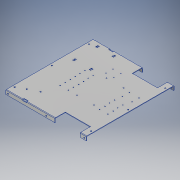
# Autodesk Inventor part: BellyPan2
Saved by Autodesk Inventor 2016 (Build 200138000, 138)
## iProperties
Created: 2017-01-21
Part Number: BellyPan2
Material: Aluminum 6061
Document SubType Name: Modeling
Designer: hamblettk
Density: 2.7 g/cm^3
Appearance: Aluminum - Flat
Author: hamblettk
Autodesk Inventor part; units mm, degrees
ref_plane "YZ Plane" through (0, 0, 0) normal (1, 0, 0) x (0, 1, 0)
ref_plane "XZ Plane" through (0, 0, 0) normal (0, 1, 0) x (-1, 0, 0)
ref_plane "XY Plane" through (0, 0, 0) normal (0, 0, 1) x (1, 0, 0)
sketch "Sketch1" plane through (0, 0, 0) normal (0, 1, 0) x (-1, 0, 0)
  line L0 (0, 0) -> (495.3, 0)
  line L1 (495.3, 0) -> (495.3, -539.75)
  line L2 (495.3, -539.75) -> (0, -539.75)
  line L3 (0, -539.75) -> (0, 0)
  dimension "d0" = 495.3
  dimension "d1" = 539.75
  constraints: 8 end point, 2 parallel, 1 horizontal, 1 perpendicular
  measures "d0" distance of L1.end L2.end
  measures "d1" distance of L0.end L1.end
extrude "Extrusion1" add sketch "Sketch1" along normal blind 3.175
sketch "Sketch2" plane through (0, 0, 0) normal (1, 0, 0) x (0, 0, -1)
  line L0 (0, 3.175) -> (0, 15.875)
  line L1 (0, 15.875) -> (3.175, 15.875)
  line L2 (3.175, 15.875) -> (3.175, 3.175)
  line L3 (0, 3.175) -> (539.75, 3.175) projected
  line L4 (3.175, 3.175) -> (0, 3.175)
  line L5 (539.75, 3.175) -> (539.75, 15.875)
  line L6 (539.75, 15.875) -> (536.575, 15.875)
  line L7 (536.575, 15.875) -> (536.575, 3.175)
  line L8 (539.75, 0) -> (539.75, 3.175) projected
  line L9 (536.575, 3.175) -> (539.75, 3.175)
  point P0 (0, 0)
  dimension "d4" = 12.7
  dimension "d5" = 3.175
  dimension "d6" = 12.7
  dimension "d7" = 3.175
  constraints: 16 end point, 5 perpendicular, 2 vertical, 1 horizontal, 1 point on line
  measures "d4" distance of L0.start L0.end
  measures "d5" distance of L0.end L1.end
  measures "d6" distance of L3.end L5.end
  measures "d7" distance of L5.end L6.end
extrude "Extrusion2" add sketch "Sketch2" against normal blind 495.3
fillet "Fillet1" radius 3.175 4 edges at (-247.65, 3.175, -536.575) (-247.65, 3.175, -3.175) (-247.65, 0, 0) (-247.65, 0, -539.75)
sketch "Sketch3" plane through (-495.3, 15.875, -539.75) normal (0, 1, 0) x (1, 0, 0)
  line L0 (495.3, 0) -> (0, 0) projected
  line L1 (495.3, 0) -> (457.2, 0)
  line L2 (457.2, 0) -> (304.8, 0)
  line L3 (304.8, 0) -> (304.8, -50.8)
  line L4 (304.8, -50.8) -> (457.2, -50.8)
  line L5 (457.2, -50.8) -> (457.2, 0)
  line L6 (0, -6.35) -> (0, -533.4) projected
  line L7 (0, -269.875) -> (495.3, -269.875)
  line L8 (495.3, -539.75) -> (0, -539.75)
  line L9 (457.2, -539.75) -> (304.8, -539.75)
  line L10 (304.8, -539.75) -> (304.8, -488.95)
  line L11 (304.8, -488.95) -> (457.2, -488.95)
  line L12 (457.2, -488.95) -> (457.2, -539.75)
  point P0 (495.3, -539.75)
  dimension "d11" = 38.1
  dimension "d12" = 152.4
  dimension "d13" = 50.8
  constraints: 22 end point, 6 symmetric about line, 4 point on line, 2 horizontal, 1 midpoint, 1 perpendicular, 1 vertical
  measures "d11" distance of L0.start L1.end
  measures "d12" distance of L1.end L2.end
  measures "d13" distance of L2.end L3.end
extrude "Extrusion3" cut sketch "Sketch3" against normal blind 495.3
sketch "Sketch5" plane through (-495.3, 15.875, -3.175) normal (0, 1, 0) x (1, 0, 0)
  line L0 (304.8, -3.175) -> (304.8, 0) projected
  line L1 (304.8, 0) -> (0, 0) projected
  line L2 (0, -3.175) -> (0, 0) projected
  line L3 (304.8, -3.175) -> (0, -3.175) projected
  line L4 (457.2, 0) -> (457.2, -3.175) projected
  line L5 (495.3, -3.175) -> (457.2, -3.175) projected
  line L6 (495.3, 0) -> (495.3, -3.175) projected
  line L7 (495.3, 0) -> (457.2, 0) projected
  line L8 (457.2, 536.575) -> (457.2, 533.4) projected
  line L9 (495.3, 533.4) -> (457.2, 533.4) projected
  line L10 (495.3, 536.575) -> (495.3, 533.4) projected
  line L11 (495.3, 536.575) -> (457.2, 536.575) projected
  line L12 (304.8, 533.4) -> (304.8, 536.575) projected
  line L13 (304.8, 536.575) -> (0, 536.575) projected
  line L14 (0, 533.4) -> (0, 536.575) projected
  line L15 (304.8, 533.4) -> (0, 533.4) projected
extrude "Extrusion4" add sketch "Sketch5" along normal blind 9.525
sketch "Sketch6" plane through (-190.5, 0, -50.8) normal (1, 0, 0) x (0, 0, -1)
  line L0 (0, 0) -> (-47.625, 0) projected
  line L1 (0, 3.175) -> (0, 0) projected
  line L2 (-44.45, 3.175) -> (0, 3.175) projected
  arc A0 (-47.625, 6.35) -> (-44.45, 3.175) centre (-44.45, 6.35) ccw projected
  line L3 (-47.625, 25.4) -> (-47.625, 6.35) projected
  line L4 (-50.8, 25.4) -> (-47.625, 25.4) projected
  line L5 (-50.8, 3.175) -> (-50.8, 25.4) projected
  arc A1 (-50.8, 3.175) -> (-47.625, 0) centre (-47.625, 3.175) ccw projected
  line L6 (485.775, 0) -> (438.15, 0) projected
  arc A2 (485.775, 0) -> (488.95, 3.175) centre (485.775, 3.175) ccw projected
  line L7 (488.95, 25.4) -> (488.95, 3.175) projected
  line L8 (485.775, 25.4) -> (488.95, 25.4) projected
  line L9 (485.775, 6.35) -> (485.775, 25.4) projected
  arc A3 (482.6, 3.175) -> (485.775, 6.35) centre (482.6, 6.35) ccw projected
  line L10 (438.15, 3.175) -> (482.6, 3.175) projected
  line L11 (438.15, 3.175) -> (438.15, 0) projected
  point P0 (-50.8, 0)
extrude "Extrusion5" cut sketch "Sketch6" against normal blind 3.175
sketch "Sketch7" plane through (-495.3, 6.35, -536.575) normal (0, 0, 1) x (1, 0, 0)
  line L0 (301.625, 0) -> (301.625, 19.05) projected
  line L1 (301.625, 9.525) -> (247.65, 9.525)
  circle A0 centre (247.65, 9.525) radius 3.5687
  point P0 (495.3, -6.35)
  dimension "d21" = 7.1374
  dimension "d22" = 53.975
  constraints: 2 end point, 1 centre point, 1 coincident, 1 horizontal, 1 midpoint
  measures "d21" diameter of A0
  measures "d22" distance from line of L0 L1.end
extrude "Extrusion6" cut sketch "Sketch7" against normal blind 3.175
sketch "Sketch8" plane through (-495.3, 6.35, -3.175) normal (0, 0, -1) x (-1, 0, 0)
  line L0 (-301.625, 19.05) -> (-301.625, 0) projected
  circle A0 centre (-247.65, 9.525) radius 3.5687
  point P0 (-495.3, -6.35)
  dimension "d26" = 7.1374
  constraints: 1 centre point
  measures "d26" diameter of A0
extrude "Extrusion7" cut sketch "Sketch8" against normal blind 3.175
sketch "Sketch9" plane through (-495.3, 6.35, -536.575) normal (0, 0, 1) x (1, 0, 0)
  line L0 (0, 0) -> (0, 19.05) projected
  line L1 (0, 9.525) -> (12.7, 9.525)
  circle A0 centre (12.7, 9.525) radius 3.5687
  point P0 (495.3, -6.35)
  dimension "d29" = 12.7
  dimension "d30" = 7.1374
  constraints: 2 end point, 1 centre point, 1 coincident, 1 horizontal, 1 midpoint
  measures "d29" distance of L1.start L1.end
  measures "d30" diameter of A0
extrude "Extrusion8" cut sketch "Sketch9" against normal blind 3.175
sketch "Sketch10" plane through (-495.3, 6.35, -3.175) normal (0, 0, -1) x (-1, 0, 0)
  line L0 (0, 0) -> (0, 19.05) projected
  line L1 (0, 9.525) -> (-12.7, 9.525)
  circle A0 centre (-12.7, 9.525) radius 3.5687
  point P0 (-495.3, -6.35)
  dimension "d33" = 12.7
  dimension "d34" = 7.1374
  constraints: 2 end point, 1 centre point, 1 coincident, 1 horizontal, 1 midpoint
  measures "d33" distance of L1.start L1.end
  measures "d34" diameter of A0
extrude "Extrusion9" cut sketch "Sketch10" against normal blind 3.175
sketch "Sketch11" plane through (0, 6.35, -3.175) normal (0, 0, -1) x (-1, 0, 0)
  line L0 (0, 0) -> (0, 19.05) projected
  line L1 (0, 9.525) -> (12.7, 9.525)
  circle A0 centre (12.7, 9.525) radius 3.5687
  point P0 (0, -6.35)
  dimension "d37" = 12.7
  dimension "d38" = 7.1374
  constraints: 2 end point, 1 centre point, 1 coincident, 1 horizontal, 1 midpoint
  measures "d37" distance of L1.start L1.end
  measures "d38" diameter of A0
extrude "Extrusion10" cut sketch "Sketch11" against normal blind 3.175
sketch "Sketch12" plane through (-38.1, 6.35, -536.575) normal (0, 0, 1) x (1, 0, 0)
  line L0 (38.1, 0) -> (0, 0) projected
  line L1 (38.1, 19.05) -> (38.1, 0) projected
  point P0 (38.1, -6.35)
  point P1 (25.3992, 9.525)
  dimension "d41" = 9.525
  dimension "d42" = 12.7008
  measures "d41" distance from line of L0 point (25.399, 9.525)
  measures "d42" distance from line of L1 point (25.399, 9.525)
hole "Hole1" at (-12.7008, 15.875, -536.575) direction (0, 0, -1) diameter 7.1374 end through all
sketch "Sketch15" plane through (0, 0, 0) normal (0, -1, 0) x (1, 0, 0)
  line L0 (-495.3, -3.175) -> (-495.3, 0) projected
  line L1 (-495.3, 0) -> (-380.1364, 0)
  line L2 (-495.3, 0) -> (-193.675, 0) projected
  line L3 (-380.1364, 0) -> (-367.4364, 0)
  line L4 (-380.1364, 0) -> (-392.8364, 0)
  line L5 (-392.8364, 0) -> (-392.8364, -9.525)
  line L6 (-392.8364, -9.525) -> (-367.4364, -9.525)
  line L7 (-367.4364, -9.525) -> (-367.4364, 0)
  line L8 (-495.3, -533.4) -> (-495.3, -6.35) projected
  line L9 (-495.3, -269.875) -> (0, -269.875)
  line L10 (-495.3, -539.75) -> (-380.1364, -539.75)
  line L11 (-495.3, -539.75) -> (-193.675, -539.75)
  line L12 (-392.8364, -539.75) -> (-392.8364, -530.225)
  line L13 (-392.8364, -530.225) -> (-367.4364, -530.225)
  line L14 (-367.4364, -530.225) -> (-367.4364, -539.75)
  point P0 (0, 0)
  dimension "d56" = 115.1636
  dimension "d57" = 12.7
  dimension "d58" = 12.7
  dimension "d59" = 9.525
  constraints: 24 end point, 7 symmetric about line, 6 point on line, 3 perpendicular, 1 horizontal, 1 midpoint
  measures "d56" distance of L0.end L1.end
  measures "d57" distance of L1.end L3.end
  measures "d58" distance of L1.end L4.end
  measures "d59" distance of L4.end L5.end
extrude "Extrusion11" cut sketch "Sketch15" against normal blind 3.175
sketch "Sketch16" plane through (0, 0, 0) normal (0, -1, 0) x (1, 0, 0)
  circle A0 centre (-12.7, -269.875) radius 3.5687
  line L0 (0, -536.575) -> (0, -3.175) projected
  line L1 (-38.1, -539.75) -> (0, -539.75) projected
  circle A1 centre (-12.7, -498.475) radius 3.5687
  circle A2 centre (-12.7, -41.275) radius 3.5687
  circle A3 centre (-482.6, -269.875) radius 3.5687
  line L2 (-495.3, -3.175) -> (-495.3, -536.575) projected
  line L3 (-495.3, -539.75) -> (-392.8364, -539.75) projected
  circle A4 centre (-482.6, -498.475) radius 3.5687
  circle A5 centre (-482.6, -41.275) radius 3.5687
  point P0 (0, 0)
  dimension "d62" = 7.1374
  dimension "d63" = 12.7
  dimension "d64" = 269.875
  dimension "d65" = 7.1374
  dimension "d66" = 12.7
  dimension "d67" = 228.6
  dimension "d68" = 7.1374
  dimension "d69" = 12.7
  dimension "d70" = 228.6
  dimension "d71" = 7.1374
  dimension "d72" = 12.7
  dimension "d73" = 269.875
  dimension "d74" = 7.1374
  dimension "d75" = 12.7
  dimension "d76" = 228.6
  dimension "d77" = 7.1374
  dimension "d78" = 12.7
  dimension "d79" = 228.6
  constraints: 6 centre point
  measures "d62" diameter of A0
  measures "d63" distance from line of L0 A0.centre
  measures "d64" distance from line of L1 A0.centre
  measures "d65" diameter of A1
  measures "d66" distance from line of L0 A1.centre
  measures "d67" distance of A0.centre A1.centre
  measures "d68" diameter of A2
  measures "d69" distance from line of L0 A2.centre
  measures "d70" distance of A0.centre A2.centre
  measures "d71" diameter of A3
  measures "d72" distance from line of L2 A3.centre
  measures "d73" distance from line of L3 A3.centre
  measures "d74" diameter of A4
  measures "d75" distance from line of L2 A4.centre
  measures "d76" distance of A3.centre A4.centre
  measures "d77" diameter of A5
  measures "d78" distance from line of L2 A5.centre
  measures "d79" distance of A3.centre A5.centre
extrude "Extrusion12" cut sketch "Sketch16" against normal blind 3.175
sketch "Sketch18" plane through (0, 3.175, 0) normal (0, -1, 0) x (1, 0, 0)
  line L0 (-392.8364, -533.4) -> (-367.4364, -533.4) projected
  line L1 (-392.8364, -539.75) -> (-392.8364, -533.4) projected
  line L2 (-392.8364, -539.75) -> (-367.4364, -539.75) projected
  line L3 (-367.4364, -533.4) -> (-367.4364, -539.75) projected
  line L4 (-367.4364, -6.35) -> (-392.8364, -6.35) projected
  line L5 (-367.4364, 0) -> (-367.4364, -6.35) projected
  line L6 (-367.4364, 0) -> (-392.8364, 0) projected
  line L7 (-392.8364, -6.35) -> (-392.8364, 0) projected
  point P0 (0, 0)
extrude "Extrusion13" cut sketch "Sketch18" against normal blind 3.175
sketch "Sketch19" plane through (-193.675, 0, -50.8) normal (0, 0, 1) x (1, 0, 0)
  line L0 (155.575, 0) -> (0, 0) projected
  line L1 (155.575, 3.175) -> (155.575, 0) projected
  line L2 (0, 3.175) -> (155.575, 3.175) projected
  line L3 (0, 3.175) -> (0, 0) projected
  point P0 (193.675, 0)
extrude "Extrusion14" cut sketch "Sketch19" against normal blind 12.7
sketch "Sketch20" plane through (-38.1, 0, -488.95) normal (0, 0, -1) x (-1, 0, 0)
  line L0 (155.575, 0) -> (0, 0) projected
  line L1 (155.575, 0) -> (155.575, 3.175) projected
  line L2 (0, 3.175) -> (155.575, 3.175) projected
  line L3 (0, 3.175) -> (0, 0) projected
  point P0 (-38.1, 0)
extrude "Extrusion15" cut sketch "Sketch20" against normal blind 12.7
sketch "Sketch21" plane through (0, 0, 0) normal (0, -1, 0) x (1, 0, 0)
  circle A0 centre (-350.8851, -350.2396) radius 2.2497
  circle A1 centre (-350.9114, -319.1371) radius 2.2497
  circle A2 centre (-350.938, -287.5981) radius 2.2497
  ellipse E0 centre (-354.1933, -225.6154) end of major axis (-352.0021, -225.6135) minor radius 2.1905
  ellipse E1 centre (-354.2089, -194.5782) end of major axis (-352.0176, -194.5764) minor radius 2.1899
  ellipse E2 centre (-303.4089, -194.5392) end of major axis (-301.2176, -194.5374) minor radius 2.1899
  ellipse E3 centre (-303.3933, -225.5744) end of major axis (-301.2021, -225.5726) minor radius 2.1905
  ellipse E4 centre (-300.1641, -256.8149) end of major axis (-302.6771, -256.817) minor radius 2.5126
  circle A3 centre (-300.138, -287.5552) radius 2.513
  circle A4 centre (-300.1114, -319.0942) radius 2.513
  circle A5 centre (-300.0851, -350.1948) radius 2.513
  circle A6 centre (-350.8851, -350.2396) radius 2.513
  circle A7 centre (-350.9114, -319.1371) radius 2.413
  circle A8 centre (-350.938, -287.5981) radius 2.513
  ellipse E5 centre (-350.9641, -256.8541) end of major axis (-348.5511, -256.8521) minor radius 2.4126
  circle A9 centre (-246.6296, -350.841) radius 2.667
  circle A10 centre (-246.9059, -168.5708) radius 2.667
  circle A11 centre (-142.512, -168.4126) radius 2.667
  circle A12 centre (-142.2357, -350.6828) radius 2.667
  ellipse E6 centre (-101.9617, -356.43) end of major axis (-104.3747, -356.43) minor radius 2.413
  ellipse E7 centre (-51.1617, -356.43) end of major axis (-53.5747, -356.43) minor radius 2.413
  ellipse E8 centre (-51.1617, -323.2691) end of major axis (-53.5747, -323.2691) minor radius 2.413
  ellipse E9 centre (-101.9617, -323.2691) end of major axis (-104.3747, -323.2691) minor radius 2.413
  ellipse E10 centre (-105.1502, -292.1816) end of major axis (-107.3414, -292.1816) minor radius 2.1913
  ellipse E11 centre (-105.1502, -261.0646) end of major axis (-107.3414, -261.0646) minor radius 2.1913
  ellipse E12 centre (-54.3502, -292.1816) end of major axis (-56.5414, -292.1816) minor radius 2.1913
  ellipse E13 centre (-54.3502, -261.0646) end of major axis (-56.5414, -261.0646) minor radius 2.1913
  circle A13 centre (-42.4909, -216.236) radius 2.5
  circle A14 centre (-101.1909, -216.2459) radius 2.5
  circle A15 centre (-100.642, -173.7423) radius 2.5
  circle A16 centre (-41.942, -173.7324) radius 2.5
  circle A17 centre (-275.3803, -143.6352) radius 1.905
  circle A18 centre (-227.6284, -143.5398) radius 1.905
  circle A19 centre (-227.7168, -100.4868) radius 1.905
  circle A20 centre (-275.4663, -100.5823) radius 1.905
  ellipse E14 centre (-434.736, -472.3219) end of major axis (-438.165, -472.3219) minor radius 3.429
  ellipse E15 centre (-377.586, -444.3819) end of major axis (-374.157, -444.3819) minor radius 3.429
  circle A21 centre (-12.6998, -269.8753) radius 3.5687
  circle A22 centre (-12.6998, -498.4753) radius 3.5685
  circle A23 centre (-12.6998, -41.2753) radius 3.5687
  line L0 (-438.5985, -28.3241) -> (-448.6768, -28.3241)
  line L1 (-448.6768, -28.3241) -> (-448.6768, -35.0231)
  spline S0 degree 4 poles (-448.6768, -35.0231) (-448.6639, -35.1127) (-448.348, -35.761) (-448.3812, -35.7746) (-448.1019, -36.3268) (-448.1852, -36.1139) (-448.2253, -36.0497) (-448.2684, -35.9471) (-448.3123, -35.8601) (-448.3471, -35.7301) (-448.3902, -35.6264) (-448.4102, -35.543) (-448.4284, -35.4842) knots 0 0 0 0 0 0.320714 0.419759 0.501148 0.569271 0.635606 0.702263 0.768643 0.834806 1 1 1 1 1
  line L2 (-448.4284, -35.4842) -> (-438.847, -35.4842)
  spline S1 degree 4 poles (-438.847, -35.4842) (-438.8355, -35.6171) (-438.8088, -35.8104) (-438.7923, -36.0459) (-438.74, -36.3561) (-438.7353, -36.5543) (-438.7189, -36.7533) (-438.7047, -36.966) (-438.6926, -37.1615) (-438.649, -37.7375) (-438.6347, -34.9543) (-438.603, -36.3425) (-438.5985, -35.0231) knots 0 0 0 0 0 0.176534 0.246794 0.316361 0.385081 0.452716 0.516863 0.592826 0.686487 1 1 1 1 1
  line L3 (-438.5985, -35.0231) -> (-438.5985, -28.3241)
  line L4 (-448.352, -20.7549) -> (-438.5985, -20.7549)
  line L5 (-448.352, -23.9299) -> (-448.352, -20.7549)
  line L6 (-438.5985, -23.9299) -> (-448.352, -23.9299)
  line L7 (-438.5985, -20.7549) -> (-438.5985, -23.9299)
  line L8 (-337.0695, -35.4845) -> (-347.0864, -35.4845)
  line L9 (-347.0864, -35.4845) -> (-347.0864, -28.3951)
  line L10 (-346.8284, -35.4842) -> (-337.247, -35.4842)
  line L11 (-337.0695, -28.3951) -> (-337.0695, -35.4845)
  ellipse E16 centre (-337.324, -28.3952) end of major axis (-337.5783, -28.3952) minor radius 0.0044 (-337.0698, -28.3951) -> (-337.3234, -28.3907) ccw
  line L12 (-346.752, -28.3907) -> (-337.3234, -28.3907)
  line L13 (-347.0768, -168.6282) -> (-336.9985, -168.6282)
  line L14 (-347.0768, -161.9292) -> (-347.0768, -168.6282)
  spline S2 degree 4 poles (-346.8284, -161.4681) (-346.8346, -161.4906) (-346.8549, -161.5222) (-346.8664, -161.5637) (-346.9192, -161.6128) (-346.9243, -161.6506) (-346.9442, -161.688) (-346.9619, -161.7261) (-346.9834, -161.7648) (-347.0156, -161.8198) (-347.0448, -161.8661) (-347.0654, -161.9031) (-347.0768, -161.9292) knots 0 0 0 0 0 0.200846 0.283365 0.365868 0.447873 0.528567 0.611335 0.696178 0.782667 1 1 1 1 1
  line L15 (-337.247, -161.4681) -> (-346.8284, -161.4681)
  spline S3 degree 4 poles (-336.9985, -161.9292) (-336.9958, -161.9015) (-336.9964, -161.863) (-337.0082, -161.8163) (-337.0309, -161.7618) (-337.0501, -161.7233) (-337.0694, -161.6844) (-337.0931, -161.647) (-337.1067, -161.6044) (-337.1672, -161.5637) (-337.1937, -161.5193) (-337.2278, -161.4909) (-337.247, -161.4681) knots 0 0 0 0 0 0.20451 0.285634 0.366889 0.448424 0.530175 0.613505 0.698082 0.783713 1 1 1 1 1
  line L16 (-336.9985, -168.6282) -> (-336.9985, -161.9292)
  line L17 (-337.0695, -176.1974) -> (-337.0695, -173.0224)
  line L18 (-346.8284, -176.1974) -> (-337.0695, -176.1974)
  line L19 (-337.0695, -173.0224) -> (-346.8284, -173.0224)
  line L20 (-346.8284, -173.0224) -> (-346.8284, -176.1974)
  line L21 (-448.6768, -168.6282) -> (-438.5985, -168.6282)
  line L22 (-438.5985, -168.6282) -> (-438.5985, -161.9292)
  line L23 (-438.847, -161.4681) -> (-448.4284, -161.4681)
  spline S4 degree 4 poles (-438.5985, -161.9292) (-438.5956, -161.9004) (-438.5959, -161.8608) (-438.608, -161.8132) (-438.6308, -161.7581) (-438.65, -161.7195) (-438.6693, -161.6806) (-438.6931, -161.6434) (-438.7067, -161.6006) (-438.767, -161.5617) (-438.7937, -161.5178) (-438.8278, -161.4904) (-438.847, -161.4681) knots 0 0 0 0 0 0.207118 0.288634 0.370017 0.451529 0.533182 0.616217 0.700347 0.785405 1 1 1 1 1
  spline S5 degree 4 poles (-448.4284, -161.4681) (-448.4341, -161.4919) (-448.4549, -161.5238) (-448.4651, -161.5678) (-448.52, -161.6151) (-448.524, -161.6549) (-448.5439, -161.6927) (-448.5612, -161.7312) (-448.5828, -161.7698) (-448.615, -161.8237) (-448.6447, -161.8682) (-448.6656, -161.9037) (-448.6768, -161.9292) knots 0 0 0 0 0 0.203146 0.286163 0.369076 0.451458 0.532565 0.615346 0.699795 0.785509 1 1 1 1 1
  line L24 (-448.6768, -161.9292) -> (-448.6768, -168.6282)
  line L25 (-448.6768, -173.0224) -> (-448.6768, -176.1974)
  line L26 (-438.5985, -173.0224) -> (-448.6768, -173.0224)
  line L27 (-448.6768, -176.1974) -> (-438.5985, -176.1974)
  line L28 (-438.5985, -176.1974) -> (-438.5985, -173.0224)
  line L29 (-347.0864, -35.4845) -> (-337.0698, -35.4845)
  line L30 (-337.0698, -35.4845) -> (-337.0698, -28.3951)
  line L31 (-337.0698, -28.3951) -> (-347.0864, -28.3951)
  line L32 (-347.0864, -28.3951) -> (-347.0864, -35.4845)
  line L33 (-448.6768, -28.3241) -> (-438.6023, -28.3241)
  line L34 (-438.6023, -28.3241) -> (-438.6023, -35.4845)
  line L35 (-438.6023, -35.4845) -> (-448.6768, -35.4845)
  line L36 (-448.6768, -35.4845) -> (-448.6768, -28.3241)
  line L37 (-438.5985, -20.7549) -> (-448.352, -20.7549)
  line L38 (-448.352, -20.7549) -> (-448.352, -23.9299)
  line L39 (-448.352, -23.9299) -> (-438.5985, -23.9299)
  line L40 (-438.5985, -23.9299) -> (-438.5985, -20.7549)
  line L41 (-337.0698, -28.3951) -> (-347.0864, -28.3951)
  line L42 (-347.0864, -28.3951) -> (-347.0864, -35.4845)
  line L43 (-347.0864, -35.4845) -> (-337.0698, -35.4845)
  line L44 (-337.0698, -35.4845) -> (-337.0698, -28.3951)
  line L45 (-347.0864, -23.9299) -> (-337.0698, -23.9299)
  line L46 (-337.0698, -23.9299) -> (-337.0698, -20.7549)
  line L47 (-337.0698, -20.7549) -> (-347.0864, -20.7549)
  line L48 (-347.0864, -20.7549) -> (-347.0864, -23.9299)
  point P0 (0, 0)
  point P1 (-448.5134, -35.4243)
  point P2 (-448.3432, -35.8171)
  point P3 (-448.2085, -36.1124)
  point P4 (-448.1481, -36.2195)
  point P5 (-448.1813, -36.1327)
  point P6 (-448.2264, -36.0413)
  point P7 (-448.2688, -35.9495)
  point P8 (-448.3089, -35.8576)
  point P9 (-448.3393, -35.7658)
  point P10 (-448.3708, -35.6724)
  point P11 (-448.4008, -35.5786)
  point P12 (-438.8246, -35.6983)
  point P13 (-438.8008, -35.9147)
  point P14 (-438.7746, -36.1347)
  point P15 (-438.7459, -36.3584)
  point P16 (-438.7328, -36.558)
  point P17 (-438.7191, -36.7585)
  point P18 (-438.7053, -36.959)
  point P19 (-438.692, -37.1576)
  point P20 (-438.6782, -37.2828)
  point P21 (-438.6501, -36.7046)
  point P22 (-438.6207, -35.8647)
  point P23 (-346.8425, -161.5026)
  point P24 (-346.8604, -161.5383)
  point P25 (-346.8836, -161.5757)
  point P26 (-346.9137, -161.6154)
  point P27 (-346.9273, -161.6509)
  point P28 (-346.9434, -161.6873)
  point P29 (-346.962, -161.7249)
  point P30 (-346.983, -161.7637)
  point P31 (-347.0065, -161.8039)
  point P32 (-347.0317, -161.8455)
  point P33 (-347.0562, -161.8879)
  point P34 (-336.9975, -161.8846)
  point P35 (-337.0033, -161.8423)
  point P36 (-337.0152, -161.8017)
  point P37 (-337.0314, -161.7622)
  point P38 (-337.05, -161.7235)
  point P39 (-337.0701, -161.6851)
  point P40 (-337.0907, -161.6468)
  point P41 (-337.1116, -161.6086)
  point P42 (-337.1475, -161.5739)
  point P43 (-337.1813, -161.5388)
  point P44 (-337.2138, -161.5034)
  point P45 (-438.5972, -161.8828)
  point P46 (-438.6031, -161.8393)
  point P47 (-438.6152, -161.7981)
  point P48 (-438.6313, -161.7584)
  point P49 (-438.65, -161.7196)
  point P50 (-438.6701, -161.6812)
  point P51 (-438.6908, -161.643)
  point P52 (-438.7117, -161.6049)
  point P53 (-438.7475, -161.5713)
  point P54 (-438.7813, -161.537)
  point P55 (-438.8138, -161.5025)
  point P56 (-448.4424, -161.5043)
  point P57 (-448.4601, -161.5412)
  point P58 (-448.4834, -161.5791)
  point P59 (-448.5138, -161.6181)
  point P60 (-448.5272, -161.6548)
  point P61 (-448.5431, -161.6922)
  point P62 (-448.5615, -161.7301)
  point P63 (-448.5825, -161.7688)
  point P64 (-448.6062, -161.8083)
  point P65 (-448.6315, -161.8485)
  point P66 (-448.6563, -161.8892)
  constraints: 98 end point, 24 centre point, 10 parallel, 5 horizontal, 5 perpendicular, 1 point on line, 115 other
extrude "Extrusion16" cut sketch "Sketch21" against normal blind 25.4 contours A2 | E0 | E1 | E2 | E3 | E4 | A3 | A4 | A5 | A6 | A7 | E5 | A9 | A10 | A11 | A12 | E6 | E7 | E8 | E9 | E10 | E11 | E12 | E13 | A13 | A14 | A15 | A16 | A17 | A18 | A19 | A20 | E14 | E15 | L34 L35 L2 S0 L1 L0 | S0 L35 L36 | L4 L7 L6 L5 | L8 L9 L31 L11 | L14 S2 L15 S3 L16 L13 | L18 L20 L19 L17 | L24 S5 L23 S4 L22 L21 | L26 L28 L27 L25 | L48 L47 L46 L45
sketch "Sketch22" plane through (-350.9114, 0, -319.1371) normal (0, -1, 0) x (1, 0, 0)
  circle A0 centre (0, 0) radius 2.2497 projected
  circle A1 centre (0.0262, -31.1025) radius 2.2497 projected
  point P0 (350.9114, 319.1371)
extrude "Extrusion17" cut sketch "Sketch22" against normal blind 25.4
body "Solid1"
